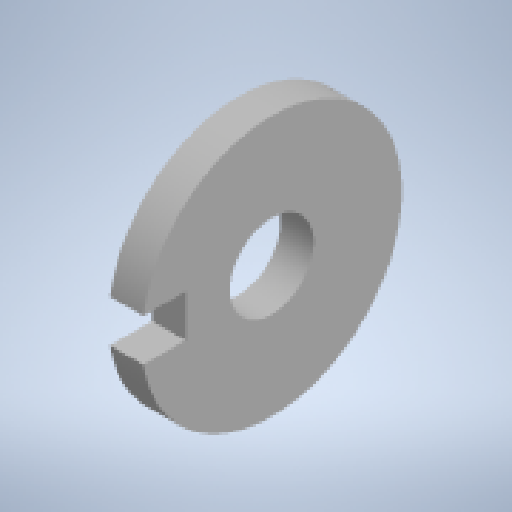
# Autodesk Inventor part: Xgantry_CableChain_bottom_connector
Saved by Autodesk Inventor 2023 (Build 270158000, 158)
## iProperties
Created: 2023-01-07
Part Number: Xgantry_CableChain_bottom_connector
Material: Generic
Document SubType Name: Modeling
Designer: a laptop
Density: 1 g/cm^3
Appearance: Default
Author: a laptop
Autodesk Inventor part; units mm, degrees
ref_plane "YZ Plane" through (0, 0, 0) normal (1, 0, 0) x (0, 1, 0)
ref_plane "XZ Plane" through (0, 0, 0) normal (0, 1, 0) x (-1, 0, 0)
ref_plane "XY Plane" through (0, 0, 0) normal (0, 0, 1) x (1, 0, 0)
sketch "Sketch1" plane through (0, 0, 0) normal (1, 0, 0) x (0, 1, 0)
  arc A0 (-1.9, 11.5447) -> (-11.7, 0) centre (0, 0) ccw
  line L0 (1.9, 11.5447) -> (1.9, 7.75)
  line L1 (1.9, 7.75) -> (-1.9, 7.75)
  line L2 (-1.9, 7.75) -> (-1.9, 11.5447)
  line L3 (0, 7.75) -> (0, 0) construction
  arc A1 (1.9, 11.5447) -> (-1.9, 11.5447) centre (0, 0) ccw construction
  circle A2 centre (0, 0) radius 3.75
  line L4 (11.7, 0) -> (11.7, -20)
  line L5 (11.7, -20) -> (-11.7, -20)
  line L6 (-11.7, -20) -> (-11.7, 0)
  arc A3 (11.7, 0) -> (1.9, 11.5447) centre (0, 0) ccw
  arc A4 (-11.7, 0) -> (11.7, 0) centre (0, 0) ccw construction
  dimension "d0" = 23.4
  dimension "d1" = 3.8
  dimension "d2" = 7.75
  dimension "d3" = 7.5
  dimension "d9" = 20
  constraints: 14 end point, 9 point on circle, 5 centre point, 3 tangent, 3 vertical, 2 coincident, 2 parallel, 2 perpendicular, 1 horizontal alignment, 1 midpoint
  measures "d0" diameter of A0
  measures "d1" distance of L0.end L1.end
  measures "d2" distance from line of point (0, 0) L1
  measures "d3" diameter of A2
  measures "d9" distance from line of L5 point (0, 0)
extrude "Extrusion1" add sketch "Sketch1" along normal blind 3
pattern_linear "Rectangular Pattern1" count 2 spacing 49.25 along (-1, 0, 0) of "Extrusion1"
sketch "Sketch2" plane through (0, 11.7, 0) normal (0, 1, 0) x (1, 0, 0)
  line L0 (-49.25, 0) -> (-49.25, 20) projected
  line L1 (-49.25, 20) -> (3.0153, 20)
  line L2 (3.0153, 20) -> (3.0153, 0)
  line L3 (3.0153, 0) -> (-49.25, 0)
  line L4 (-49.25, 0) -> (-49.25, 20)
  constraints: 8 end point, 2 parallel, 1 horizontal, 1 perpendicular
extrude "Extrusion2" add sketch "Sketch2" along normal blind 3
sketch "Sketch3" plane through (0, -11.7, -20) normal (0, -1, 0) x (1, 0, 0)
  line L0 (-49.25, 0) -> (-46.25, 0) projected
  line L1 (-49.25, 0) -> (3, 0)
  line L2 (3, 0) -> (3, 26)
  line L3 (3, 26) -> (-49.25, 26)
  line L4 (-49.25, 26) -> (-49.25, 0)
  point P0 (0, 20)
  dimension "d12" = 6
  constraints: 8 end point, 2 parallel, 1 coincident, 1 horizontal, 1 perpendicular
  measures "d12" distance from line of point (0, 20) L3
extrude "Extrusion3" add sketch "Sketch3" along normal blind 3
sketch "Sketch4" plane through (0, -11.7, -20) normal (0, 1, 0) x (1, 0, 0)
  line L0 (-46.25, -31.5447) -> (-46.25, -20) construction
  line L1 (-46.25, -20) -> (-49.25, -20)
  line L2 (-49.25, -20) -> (-49.25, -26)
  line L3 (-49.25, -26) -> (-46.25, -26)
  line L4 (-46.25, -26) -> (-46.25, -20)
  line L5 (0, -20) -> (0, 0) construction
  line L6 (3, -26) -> (-49.25, -26) construction
  line L7 (0, -20) -> (3, -20)
  line L8 (3, -20) -> (3, -26)
  line L9 (3, -26) -> (0, -26)
  line L10 (0, -26) -> (0, -20)
  constraints: 16 end point, 4 parallel, 2 horizontal, 2 perpendicular
extrude "Extrusion4" add sketch "Sketch4" along normal up to surface round surface about axis through (-49.25, 0, 0) along (1, 0, 0) radius 11.7 far side no
sketch "Sketch5" plane through (-46.25, 11.7, 0) normal (0, 0, 1) x (1, 0, 0)
  line L0 (-3, 0) -> (0, 0) projected
  line L1 (0, 0) -> (46.25, 0) projected
  line L2 (46.25, 0) -> (49.25, 0) projected
  line L3 (49.25, 0) -> (49.2653, 0) projected
  line L4 (49.2653, 0) -> (49.2653, 3) projected
  line L5 (-3, 3) -> (49.2653, 3) projected
  line L6 (-3, 0) -> (-3, 3) projected
  point P0 (46.25, -11.7)
extrude "Extrusion5" add sketch "Sketch5" along normal blind 30
sketch "Sketch6" plane through (0, 11.7, 0) normal (0, -1, 0) x (1, 0, 0)
  line L0 (0, -20) -> (0, 0) construction
  line L1 (3.0153, 30) -> (3.0153, -20) construction
  line L2 (0, 0) -> (3.0153, 0)
  line L3 (3.0153, 0) -> (3.0153, 2)
  line L4 (3.0153, 2) -> (0, 2)
  line L5 (0, 2) -> (0, 0)
  line L6 (-46.25, -20) -> (-46.25, 0) construction
  line L7 (-49.25, 0) -> (-49.25, 30) construction
  line L8 (-46.25, 0) -> (-49.25, 0)
  line L9 (-49.25, 0) -> (-49.25, 2)
  line L10 (-49.25, 2) -> (-46.25, 2)
  line L11 (-46.25, 2) -> (-46.25, 0)
  dimension "d19" = 2
  constraints: 16 end point, 4 parallel, 3 point on line, 2 horizontal, 2 perpendicular
  measures "d19" distance from line of L2.end L4
extrude "Extrusion6" add sketch "Sketch6" along normal up to surface round surface about axis through (0, 0, 0) along (1, 0, 0) radius 11.7 far side no
sketch "Sketch7" plane through (0, -14.7, -20) normal (0, -1, 0) x (1, 0, 0)
  circle A0 centre (-38.125, 10) radius 2.8812
  circle A1 centre (-8.125, 10) radius 2.8812
  line L0 (-49.25, 0) -> (3, 0) construction
  line L1 (-38.125, 10) -> (-8.125, 10) construction
  line L2 (-23.125, 10) -> (-23.125, 0) construction
  line L3 (-46.25, 0) -> (0, 0) construction
  point P0 (0, 20)
  dimension "d22" = 5.7625
  dimension "d23" = 30
  dimension "d24" = 10
  constraints: 4 end point, 2 centre point, 2 midpoint, 1 equal radius, 1 horizontal, 1 horizontal alignment, 1 perpendicular
  measures "d22" diameter of A0
  measures "d23" distance of L1.start L1.end
  measures "d24" distance of L2.start L2.end
extrude "Extrusion7" cut sketch "Sketch7" against normal up to surface (29.4 mm away)
body "Solid1"
